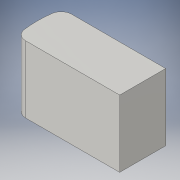
# Autodesk Inventor part: Button
Saved by Autodesk Inventor 2016 (Build 200138000, 138)
## iProperties
Created: 2016-05-07
Part Number: Button
Material: ABS Plastic
Document SubType Name: Modeling
Designer: agmle
Density: 1.06 g/cm^3
Appearance: Smooth - White
Mass: 0.0723943 g
Surface Area: 1.04027 cm^2
Volume: 0.0682965 cm^3
Author: agmle
Autodesk Inventor part; units mm, degrees
ref_plane "YZ Plane" through (0, 0, 0) normal (1, 0, 0) x (0, 1, 0)
ref_plane "XZ Plane" through (0, 0, 0) normal (0, 1, 0) x (-1, 0, 0)
ref_plane "XY Plane" through (0, 0, 0) normal (0, 0, 1) x (1, 0, 0)
sketch "Sketch1" plane through (0, 0, 0) normal (0, 1, 0) x (-1, 0, 0)
  line L0 (0, 0) -> (6.15, 0)
  line L1 (6.15, 0) -> (6.15, -2.75) construction
  line L2 (6.15, -2.75) -> (0, -2.75)
  line L3 (0, -2.75) -> (0, 0)
  arc A0 (6.15, -2.75) -> (6.15, 0) centre (-0.0771, -1.375) ccw
  line L4 (-0.0771, 0) -> (-0.0771, -2.75) construction
  line L5 (6.3, 0.5033) -> (6.3, -3.5493) construction
  dimension "d0" = 2.75
  dimension "d1" = 6.3
  dimension "d2" = 6.15
  constraints: 12 end point, 3 parallel, 2 perpendicular, 2 point on circle, 2 point on line, 1 centre point, 1 coincident, 1 horizontal, 1 midpoint, 1 tangent
  measures "d0" distance between parallel lines of L2 L0
  measures "d1" distance between parallel lines of L3 L5
  measures "d2" distance between parallel lines of L3 L1
extrude "Extrusion1" add sketch "Sketch1" along normal blind 4
fillet "Fillet1" radius 0.625 2 edges at (-6.15, 2, -2.75) (-6.15, 2, 0)
body "Solid1"
